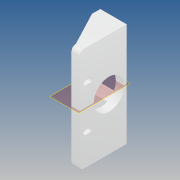
# Autodesk Inventor part: 3223_Motor Bracket_V1
Saved by Autodesk Inventor 2020 (Build 240168000, 168)
## iProperties
Created: 2020-01-12
Part Number: 3223_Motor Bracket_V1
Material: Aluminum 6061
Document SubType Name: Modeling
Designer: MPI
Density: 2.7 g/cm^3
Appearance: Aluminum - Flat
Author: MPI
Autodesk Inventor part; units mm, degrees
ref_plane "YZ Plane" through (0, 0, 0) normal (1, 0, 0) x (0, 1, 0)
ref_plane "XZ Plane" through (0, 0, 0) normal (0, 1, 0) x (-1, 0, 0)
ref_plane "XY Plane" through (0, 0, 0) normal (0, 0, 1) x (1, 0, 0)
sketch "Sketch1" plane through (0, 0, 0) normal (0, 0, 1) x (1, 0, 0)
  line L0 (54.5, 1) -> (0, 1) construction
  line L1 (54.5, 1) -> (54.5, 89) construction
  line L2 (32.5, 89) -> (54.5, 89) construction
  line L3 (32.5, 97) -> (32.5, 89) construction
  line L4 (32.5, 97) -> (21.5, 97) construction
  line L5 (21.5, 97) -> (21.5, 139.7) construction
  line L6 (21.5, 139.7) -> (32.5, 139.7) construction
  line L7 (32.5, 147.7) -> (32.5, 139.7) construction
  line L8 (54.5, 147.7) -> (32.5, 147.7) construction
  line L9 (54.5, 147.7) -> (54.5, 225) construction
  line L10 (54.5, 225) -> (37.3185, 225) construction
  ellipse E0 centre (35.382, 226) end of major axis (37.618, 226) minor radius 2 (35.382, 224) -> (37.3185, 225) ccw construction
  line L11 (0, 224) -> (35.382, 224) construction
  line L12 (0, 1) -> (0, 224) construction
  line L13 (19.5, 108.15) -> (19.5, 128.15) construction
  line L14 (21.5, 130.15) -> (21.5, 106.15) construction
  line L15 (21.5, 106.15) -> (18.4151, 106.15) construction
  line L16 (18.4151, 106.15) -> (18.4151, 131.388) construction
  line L17 (18.4151, 131.388) -> (21.5, 131.388) construction
  line L18 (21.5, 131.388) -> (21.5, 106.15) construction
  line L19 (15.5, 80.65) -> (21.5, 80.65)
  line L20 (21.5, 80.65) -> (21.5, 155.65)
  line L21 (21.5, 155.65) -> (15.5, 155.65)
  line L22 (15.5, 155.65) -> (15.5, 80.65)
  point P0 (0, 0)
  point P1 (15.5, 118.15)
  point P2 (19.5, 118.15)
  dimension "d0" = 75
  dimension "d1" = 6
  constraints: 16 end point, 4 parallel, 2 horizontal, 2 midpoint, 2 perpendicular, 1 horizontal alignment, 1 point on line, 1 other
  measures "d0" distance of L21.end L19.start
  measures "d1" distance of L19.start L19.end
ref_plane "Work Plane1" through (21.5, 100, 33.9) normal (0, 0, 1) x (1, 0, 0)
extrude "Extrusion1" add sketch "Sketch1" along normal up to surface (33.9 mm away)
sketch "Sketch2" plane through (15.5, 80.65, 0) normal (-1, 0, 0) x (0, 0, 1)
  circle A0 centre (28.25, 22) radius 1.5 projected
  circle A1 centre (28.25, 53) radius 1.5 projected
  line L0 (29.75, 22) -> (26.75, 22) construction
  line L1 (29.75, 20.5) -> (26.75, 20.5)
  line L2 (26.75, 23.5) -> (29.75, 23.5)
  arc A2 (29.75, 20.5) -> (29.75, 23.5) centre (29.75, 22) ccw
  arc A3 (26.75, 23.5) -> (26.75, 20.5) centre (26.75, 22) ccw
  line L3 (29.75, 53) -> (26.75, 53) construction
  line L4 (29.75, 51.5) -> (26.75, 51.5)
  line L5 (26.75, 54.5) -> (29.75, 54.5)
  arc A4 (29.75, 51.5) -> (29.75, 54.5) centre (29.75, 53) ccw
  arc A5 (26.75, 54.5) -> (26.75, 51.5) centre (26.75, 53) ccw
  point P0 (0, -80.65)
  constraints: 16 end point, 8 point on circle, 8 tangent, 4 centre point, 3 parallel, 2 horizontal alignment, 2 midpoint, 1 horizontal, 2 other
extrude "Extrusion2" cut sketch "Sketch2" against normal through all
fillet "Fillet1" radius 3.175 2 edges at (18.5, 80.65, 33.9) (18.5, 155.65, 33.9)
sketch "Sketch3" plane through (15.5, 80.65, 0) normal (0, -1, 0) x (1, 0, 0)
  line L0 (0, 0) -> (6, 0) projected
  line L1 (0, 0) -> (-13.05, 0)
  line L2 (-13.05, 0) -> (-13.05, 6)
  line L3 (-13.05, 6) -> (0, 6)
  line L4 (0, 6) -> (0, 0)
  line L5 (13.8, -11) -> (39, -11) projected
  line L6 (39, -1) -> (39, -11) projected
  line L7 (-15.5, -1) -> (39, -1) projected
  line L8 (-15.5, -2.18) -> (-15.5, -1) projected
  line L9 (-15.5, -2.18) -> (-11.3, -2.18) projected
  line L10 (-11.3, -10.45) -> (-11.3, -2.18) projected
  arc A0 (-11.3, -10.45) -> (-10.0386, -11.1035) centre (-10.5, -10.45) ccw projected
  line L11 (-3.0921, -6.1997) -> (-10.0386, -11.1035) projected
  arc A1 (-1.2, -7.18) -> (-3.0921, -6.1997) centre (-2.4, -7.18) ccw projected
  line L12 (-1.2, -37.82) -> (-1.2, -7.18) projected
  arc A2 (-3.0921, -38.8003) -> (-1.2, -37.82) centre (-2.4, -37.82) ccw projected
  line L13 (-10.0386, -33.8965) -> (-3.0921, -38.8003) projected
  arc A3 (-10.0386, -33.8965) -> (-11.3, -34.55) centre (-10.5, -34.55) ccw projected
  line L14 (-11.3, -42.82) -> (-11.3, -34.55) projected
  line L15 (-11.3, -42.82) -> (-15.5, -42.82) projected
  line L16 (-15.5, -44) -> (-15.5, -42.82) projected
  line L17 (39, -44) -> (-15.5, -44) projected
  line L18 (39, -34) -> (39, -44) projected
  line L19 (39, -34) -> (13.8, -34) projected
  line L20 (13.8, -34) -> (13.8, -11) projected
  line L21 (6, 0) -> (6, 30.725) projected
  point P0 (-15.5, 0)
  point P1 (-13.05, 3)
  dimension "d8" = 6
  dimension "d17" = 19.05
  constraints: 8 end point, 2 parallel, 1 horizontal, 1 midpoint, 1 perpendicular
  measures "d8" distance of L1.end L2.end
  measures "d17" distance between parallel lines of L21 L2
extrude "Extrusion3" add sketch "Sketch3" against normal up to surface (75 mm away) contours L1 L2 L3 L4
sketch "Sketch4" plane through (2.45, 80.65, 0) normal (-1, 0, 0) x (0, 0, 1)
  circle A0 centre (12.75, 37.5) radius 2.5 projected
  line L0 (6, 0) -> (6, 75) projected
  circle A1 centre (12.75, 37.5) radius 12.75
  line L1 (0, 0) -> (0, 75) projected
  circle A2 centre (12.75, 37.5) radius 13.75
  point P0 (0, -80.65)
  point P1 (6, 48.3167)
  point P2 (6, 26.6833)
  point P3 (6, 25.5209)
  point P4 (6, 49.4791)
  dimension "d13" = 1
  constraints: 2 centre point, 2 coincident, 1 tangent
  measures "d13" radial gap between concentric circles of A1 A2
extrude "Extrusion4" cut sketch "Sketch4" against normal up to surface (13.05 mm away) contours A2 L1 A1 L0 | A1 L0 | A2 L1 | A1 L1 A2 L0 picked at (3.6647, 36.3512)
fillet "Fillet2" radius 1.016 2 edges at (8.975, 113.0022, 0) (8.975, 123.2978, 0)
sketch "Sketch5" plane through (15.5, 83.825, 33.9) normal (-1, 0, 0) x (0, 0, 1)
  circle A0 centre (-21.15, 34.325) radius 11 projected
  point P0 (-33.9, -83.825)
extrude "Extrusion5" cut sketch "Sketch5" against normal through all
sketch "Sketch6" plane through (15.5, 80.65, 30.725) normal (0, -1, 0) x (1, 0, 0)
  line L0 (0, 0) -> (6, 0) projected
  line L1 (0, -24.725) -> (0, 0) projected
  line L2 (0, -24.725) -> (-13.05, -24.725) projected
  line L3 (-13.05, -24.725) -> (-13.05, -30.725) projected
  line L4 (-13.05, -30.725) -> (6, -30.725) projected
  line L5 (6, -30.725) -> (6, 0) projected
  line L6 (0, -24.725) -> (-13.05, -24.725) projected
  line L7 (0, 0) -> (0, 3.175) projected
  line L8 (-13.05, -24.725) -> (0, 0)
  point P0 (-15.5, -30.725)
  constraints: 2 end point
extrude "Extrusion6" add sketch "Sketch6" against normal blind 5 contours L1 L2 L8
fillet "Fillet3" radius 1.016 5 edges at (8.975, 85.65, 6) (15.5, 85.65, 18.3625) (15.5, 95.9104, 6) (15.5, 110.1487, 0.6905) (15.5, 107.7746, 3.727)
sketch "Sketch7" plane through (2.45, 106.1709, 6) normal (0, 0, 1) x (1, 0, 0)
  line L0 (12.034, 0) -> (12.034, -19.5049) construction
  line L1 (12.034, 0) -> (0, 0) construction
  line L2 (0, -19.5049) -> (0, 0) construction
  line L3 (12.034, -19.5049) -> (0, -19.5049) construction
  line L4 (0, -25.5209) -> (0, -19.5049) construction
  line L5 (0, -19.5049) -> (12.034, 0) construction
  circle A0 centre (6.017, -9.7524) radius 1.5875
  point P0 (-2.45, -106.1709)
  dimension "d21" = 3.175
  constraints: 2 end point, 1 centre point, 1 midpoint
  measures "d21" diameter of A0
extrude "Extrusion7" cut sketch "Sketch7" against normal through all
ref_plane "Work Plane2" through (21.5, 118.15, 0) normal (0, -1, 0) x (1, 0, 0)
mirror "Mirror1" about plane through (21.5, 118.15, 0) normal (0, -1, 0) of "Extrusion6", "Extrusion7"
fillet "Fillet4" radius 1.016 7 edges at (15.5, 126.1513, 0.6905) (15.5, 128.5254, 3.727) (15.5, 140.3896, 6) (8.975, 150.65, 6) (15.5, 150.65, 18.3625) (15.5, 153.15, 30.725) (15.5, 83.658, 30.725)
body "Solid1"
